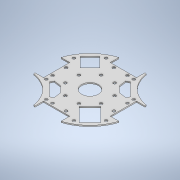
# Autodesk Inventor part: motherBoard_ыефтв
Saved by Autodesk Inventor 2020 (Build 240168000, 168)
## iProperties
Created: 2024-09-19
Part Number: motherBoard_ыефтв
Material: Типовые
Document SubType Name: Modeling
Designer: Ivan
Density: 1 g/cm^3
Appearance: По умолчанию
Author: Ivan
Autodesk Inventor part; units mm, degrees
ref_plane "YZ Plane" through (0, 0, 0) normal (1, 0, 0) x (0, 1, 0)
ref_plane "XZ Plane" through (0, 0, 0) normal (0, 1, 0) x (-1, 0, 0)
ref_plane "XY Plane" through (0, 0, 0) normal (0, 0, 1) x (1, 0, 0)
sketch "Эскиз3" plane through (0, 0, 0) normal (0, 1, 0) x (-1, 0, 0)
  line L0 (-54.5982, 80.4592) -> (-22.4528, 48.3138)
  line L1 (-22.4528, 48.3138) -> (-48.3138, 22.4528)
  line L2 (-48.3138, 22.4528) -> (-80.4592, 54.5982)
  line L3 (-80.4592, 54.5982) -> (-54.5982, 80.4592)
  line L4 (32.5269, -55.8614) -> (55.8614, -32.5269)
  line L5 (55.8614, -32.5269) -> (79.196, -55.8614)
  line L6 (79.196, -55.8614) -> (55.8614, -79.196)
  line L7 (55.8614, -79.196) -> (32.5269, -55.8614)
  circle A0 centre (0, 0) radius 20
  circle A1 centre (16, -72.43) radius 1.5
  circle A2 centre (16, -42.22) radius 1.5
  circle A3 centre (42.22, -16) radius 1.5
  circle A4 centre (42.22, 16) radius 1.5
  circle A5 centre (72.43, 31) radius 1.5
  circle A6 centre (-44.87, 82.9015) radius 1.5
  circle A7 centre (31, 72.43) radius 1.5
  circle A8 centre (72.43, 16) radius 1.5
  circle A9 centre (-42.22, 16) radius 1.5
  circle A10 centre (-42.22, -16) radius 1.5
  circle A11 centre (-16, -42.22) radius 1.5
  circle A12 centre (-16, -72.43) radius 1.5
  circle A13 centre (-72.43, -31) radius 1.5
  circle A14 centre (72.43, -16) radius 1.5
  circle A15 centre (16, 42.22) radius 1.5
  circle A16 centre (-82.9015, 44.87) radius 1.5
  circle A17 centre (-16, 72.43) radius 1.5
  circle A18 centre (44.87, -82.9015) radius 1.5
  circle A19 centre (16, 72.43) radius 1.5
  circle A20 centre (-16, 42.22) radius 1.5
  circle A21 centre (-72.43, 16) radius 1.5
  circle A22 centre (-72.43, -16) radius 1.5
  circle A23 centre (-31, -72.43) radius 1.5
  circle A24 centre (82.9015, -44.87) radius 1.5
  arc A25 (-34.57, -98.0863) -> (-98.0863, -34.57) centre (-109.0212, -109.0212) ccw
  arc A26 (-34.57, -98.0863) -> (-31, -99.2724) centre (0, 0) ccw
  line L8 (-31, -99.2724) -> (-31, -78.7724)
  line L9 (-31, -78.7724) -> (31, -78.7724)
  line L10 (31, -78.7724) -> (31, -99.2724)
  arc A27 (31, -99.2724) -> (99.2724, -31) centre (0, 0) ccw
  line L11 (99.2724, -31) -> (78.7724, -31)
  line L12 (78.7724, -31) -> (78.7724, 31)
  line L13 (78.7724, 31) -> (99.2724, 31)
  arc A28 (99.2724, 31) -> (98.0863, 34.57) centre (0, 0) ccw
  arc A29 (34.57, 98.0863) -> (98.0863, 34.57) centre (109.0212, 109.0212) ccw
  arc A30 (34.57, 98.0863) -> (31, 99.2724) centre (0, 0) ccw
  line L14 (31, 99.2724) -> (31, 78.7724)
  line L15 (31, 78.7724) -> (-31, 78.7724)
  line L16 (-31, 78.7724) -> (-31, 99.2724)
  arc A31 (-31, 99.2724) -> (-99.2724, 31) centre (0, 0) ccw
  line L17 (-99.2724, 31) -> (-78.7724, 31)
  line L18 (-78.7724, 31) -> (-78.7724, -31)
  line L19 (-78.7724, -31) -> (-99.2724, -31)
  arc A32 (-99.2724, -31) -> (-98.0863, -34.57) centre (0, 0) ccw
  constraints: 40 end point, 33 centre point, 16 point on circle
extrude "Выдавливание1" add sketch "Эскиз3" along normal blind 2.66
sketch "Эскиз5" plane through (0, 2.66, 0) normal (0, 1, 0) x (1, 0, 0)
  line L0 (31, 78.7724) -> (-31, 78.7724) projected
  line L1 (-31, 78.7724) -> (-31, 99.2724) projected
  arc A0 (-31, 99.2724) -> (-99.2724, 31) centre (0, 0) ccw projected
  line L2 (-99.2724, 31) -> (-78.7724, 31) projected
  line L3 (-78.7724, 31) -> (-78.7724, -31) projected
  line L4 (-78.7724, -31) -> (-99.2724, -31) projected
  arc A1 (-99.2724, -31) -> (-98.0863, -34.57) centre (0, 0) ccw projected
  arc A2 (-34.57, -98.0863) -> (-98.0863, -34.57) centre (-109.0212, -109.0212) ccw projected
  arc A3 (-34.57, -98.0863) -> (-31, -99.2724) centre (0, 0) ccw projected
  line L5 (-31, -99.2724) -> (-31, -78.7724) projected
  line L6 (-31, -78.7724) -> (31, -78.7724) projected
  line L7 (31, -78.7724) -> (31, -99.2724) projected
  arc A4 (31, -99.2724) -> (99.2724, -31) centre (0, 0) ccw projected
  line L8 (99.2724, -31) -> (78.7724, -31) projected
  line L9 (78.7724, -31) -> (78.7724, 31) projected
  line L10 (78.7724, 31) -> (99.2724, 31) projected
  arc A5 (99.2724, 31) -> (98.0863, 34.57) centre (0, 0) ccw projected
  arc A6 (34.57, 98.0863) -> (98.0863, 34.57) centre (109.0212, 109.0212) ccw projected
  arc A7 (34.57, 98.0863) -> (31, 99.2724) centre (0, 0) ccw projected
  line L11 (31, 99.2724) -> (31, 78.7724) projected
  circle A8 centre (31, 72.43) radius 1.5 projected
  circle A9 centre (72.43, -16) radius 1.5 projected
  circle A10 centre (-16, -72.43) radius 1.5 projected
  circle A11 centre (-16, -42.22) radius 1.5 projected
  circle A12 centre (72.43, 31) radius 1.5 projected
  circle A13 centre (16, 42.22) radius 1.5 projected
  circle A14 centre (42.22, -16) radius 1.5 projected
  circle A15 centre (0, 0) radius 20 projected
  circle A16 centre (-16, 72.43) radius 1.5 projected
  circle A17 centre (-16, 42.22) radius 1.5 projected
  circle A18 centre (-42.22, 16) radius 1.5 projected
  circle A19 centre (-42.22, -16) radius 1.5 projected
  circle A20 centre (-72.43, -31) radius 1.5 projected
  circle A21 centre (-31, -72.43) radius 1.5 projected
  circle A22 centre (-72.43, -16) radius 1.5 projected
  circle A23 centre (42.22, 16) radius 1.5 projected
  circle A24 centre (16, 72.43) radius 1.5 projected
  circle A25 centre (-72.43, 16) radius 1.5 projected
  circle A26 centre (16, -72.43) radius 1.5 projected
  circle A27 centre (16, -42.22) radius 1.5 projected
  circle A28 centre (72.43, 16) radius 1.5 projected
  circle A29 centre (82.9015, -44.87) radius 1.5 projected
  circle A30 centre (-82.9015, 44.87) radius 1.5 projected
  circle A31 centre (-44.87, 82.9015) radius 1.5 projected
  circle A32 centre (44.87, -82.9015) radius 1.5 projected
  line L12 (-55.8614, 32.5269) -> (-79.196, 55.8614) projected
  line L13 (-79.196, 55.8614) -> (-55.8614, 79.196) projected
  line L14 (-55.8614, 79.196) -> (-32.5269, 55.8614) projected
  line L15 (-32.5269, 55.8614) -> (-55.8614, 32.5269) projected
  line L16 (48.3138, -22.4528) -> (80.4592, -54.5982) projected
  line L17 (80.4592, -54.5982) -> (54.5982, -80.4592) projected
  line L18 (54.5982, -80.4592) -> (22.4528, -48.3138) projected
  line L19 (22.4528, -48.3138) -> (48.3138, -22.4528) projected
  circle A33 centre (-31, -72.43) radius 3.3
  circle A34 centre (-16, -72.43) radius 3.3
  circle A35 centre (-16, -42.22) radius 1.5 projected
  circle A36 centre (-16, -42.22) radius 3.3
  circle A37 centre (-42.22, -16) radius 1.5 projected
  circle A38 centre (-42.22, -16) radius 3.3
  circle A39 centre (-42.22, 16) radius 3.3
  circle A40 centre (-72.43, -31) radius 1.5 projected
  circle A41 centre (-72.43, -31) radius 3.3
  circle A42 centre (-72.43, -16) radius 1.5 projected
  circle A43 centre (-72.43, -16) radius 3.3
  circle A44 centre (-72.43, 16) radius 1.5 projected
  circle A45 centre (-72.43, 16) radius 3.3
  circle A46 centre (-16, 42.22) radius 1.5 projected
  circle A47 centre (-16, 42.22) radius 3.3
  circle A48 centre (16, 42.22) radius 1.5 projected
  circle A49 centre (16, 42.22) radius 3.3
  circle A50 centre (42.22, 16) radius 1.5 projected
  circle A51 centre (42.22, 16) radius 3.3
  circle A52 centre (42.22, -16) radius 1.5 projected
  circle A53 centre (42.22, -16) radius 3.3
  circle A54 centre (16, -42.22) radius 1.5 projected
  circle A55 centre (16, -42.22) radius 3.3
  circle A56 centre (16, -72.43) radius 1.5 projected
  circle A57 centre (16, -72.43) radius 3.3
  circle A58 centre (44.87, -82.9015) radius 1.5 projected
  circle A59 centre (44.87, -82.9015) radius 3.3
  circle A60 centre (82.9015, -44.87) radius 1.5 projected
  circle A61 centre (82.9015, -44.87) radius 3.3
  circle A62 centre (72.43, -16) radius 3.3
  circle A63 centre (72.43, 16) radius 1.5 projected
  circle A64 centre (72.43, 16) radius 3.3
  circle A65 centre (72.43, 31) radius 1.5 projected
  circle A66 centre (72.43, 31) radius 3.3
  circle A67 centre (31, 72.43) radius 3.3
  circle A68 centre (16, 72.43) radius 1.5 projected
  circle A69 centre (16, 72.43) radius 3.3
  circle A70 centre (-82.9015, 44.87) radius 3.3
  circle A71 centre (-44.87, 82.9015) radius 3.3
  circle A72 centre (-16, 72.43) radius 1.5 projected
  circle A73 centre (-16, 72.43) radius 3.3
  line L20 (-55.8614, 32.5269) -> (-79.196, 55.8614) projected
  dimension "d2" = 6.6
  constraints: 24 centre point, 24 coincident, 23 equal radius
  measures "d2" diameter of A33
extrude "Выдавливание2" cut sketch "Эскиз5" against normal blind 2.66 contours A8 | A9 | A11 | A12 | A13 | A14 | A16 | A17 | A18 | A19 | A21 | A23 | A24 | A25 | A26 | A27 | A28 | A29 | A30 | A31 | A32 | A33 | A34 | A36 | A38 | A39 | A41 | A43 | A45 | A47 | A49 | A51 | A53 | A55 | A57 | A59 | A61 | A62 | A64 | A66 | A67 | A69 | A70 | A71 | A73
sketch "Эскиз6" plane through (0, 2.66, 0) normal (0, 1, 0) x (1, 0, 0)
  circle A0 centre (-72.43, -31) radius 3.3 construction
  circle A1 centre (-72.43, -16) radius 3.3 construction
  circle A2 centre (-31, -72.43) radius 3.3 construction
  circle A3 centre (-16, -72.43) radius 3.3 construction
  line L0 (-72.43, -31) -> (-72.43, -16) construction
  line L1 (-31, -72.43) -> (-16, -72.43) construction
  line L2 (-32.6924, -63.2376) -> (-63.2376, -32.6924)
  circle A4 centre (-16, -42.22) radius 3.3 construction
  circle A5 centre (-42.22, -16) radius 3.3 construction
  line L3 (-16, -42.22) -> (-42.22, -16) construction
  line L4 (-42.0023, -27.4404) -> (-59.5377, -25.1696)
  line L5 (-27.4404, -42.0023) -> (-25.1696, -59.5377)
  line L6 (-63.2376, -32.6924) -> (-59.5377, -25.1696) construction
  line L7 (-32.6924, -63.2376) -> (-25.1696, -59.5377) construction
  line L8 (-27.4404, -42.0023) -> (-42.0023, -27.4404) construction
  line L9 (-27.4404, -42.0023) -> (-42.0023, -27.4404)
  line L10 (-59.5377, -25.1696) -> (-63.2376, -32.6924)
  line L11 (-32.6924, -63.2376) -> (-25.1696, -59.5377)
  line L12 (32.6924, 63.2376) -> (63.2376, 32.6924)
  line L13 (42.0023, 27.4404) -> (59.5377, 25.1696)
  line L14 (63.2376, 32.6924) -> (59.5377, 25.1696)
  line L15 (32.6924, 63.2376) -> (25.1696, 59.5377)
  line L16 (27.4404, 42.0023) -> (25.1696, 59.5377)
  line L17 (27.4404, 42.0023) -> (42.0023, 27.4404)
  point P0 (0, 0)
  point P1 (-23.5, -72.43)
  point P2 (-72.43, -23.5)
  point P3 (-29.11, -29.11)
  point P4 (72.43, 23.5)
  point P5 (23.5, 72.43)
  point P6 (29.11, 29.11)
  dimension "d7" = 13
  dimension "d8" = 13
  dimension "d9" = 13
  dimension "d10" = 13
  dimension "d11" = 13
  dimension "d12" = 13
  dimension "d15" = 360
  constraints: 36 end point, 12 point on line, 3 midpoint, 2 collinear, 1 horizontal, 1 vertical, 31 other
  measures "d7" distance of L2.end point (-72.43, -23.5)
  measures "d8" distance of L4.end point (-72.43, -23.5)
  measures "d9" distance of L2.start point (-23.5, -72.43)
  measures "d10" distance of L5.end point (-23.5, -72.43)
  measures "d11" distance of L5.start point (-29.11, -29.11)
  measures "d12" distance of L4.start point (-29.11, -29.11)
extrude "Выдавливание3" cut sketch "Эскиз6" against normal blind 2.66
equation "\"d8\" = d7"
equation "\"d9\" = d7"
equation "\"d10\" = d9"
equation "\"d11\" = d7"
equation "\"d12\" = d11"
